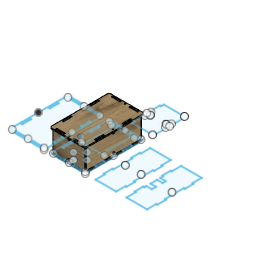
final l final v1 (Autodesk Fusion 360 design; units mm, degrees)
Autodesk Fusion 360 part; units mm, degrees
sketch "Sketch1" plane through (0, 0, 0) normal (0, 0, 1) x (1, 0, 0)
  line L0 (180, 78.114) -> (177.2, 78.114)
  line L1 (90, 52.114) -> (90, 78.114)
  line L2 (90, 81.114) -> (90, 107.114)
  line L3 (177.2, 76.484) -> (174.45, 76.484)
  line L4 (-89.654, 3.2) -> (-89.654, 6.6)
  line L5 (84.45, 76.484) -> (84.45, 78.114)
  arc A0 (-5, 0) -> (0, 5) centre (-5, 5) ccw
  line L6 (-64.654, 6.6) -> (-64.654, 3.2)
  line L7 (180, 0) -> (180, 27.114)
  line L8 (37, 78.114) -> (37, 79.614)
  line L9 (35.55, 76.484) -> (35.55, 78.114)
  line L10 (120, 27.114) -> (120, 0)
  line L11 (183.2, 52.114) -> (180, 52.114)
  circle A1 centre (-17.936, 73.3627) radius 1.5
  circle A2 centre (-4.7, 86.2139) radius 1.7
  line L12 (183.2, 27.114) -> (183.2, 52.114)
  line L13 (37, 81.114) -> (37, 79.614)
  line L14 (87.2, 76.484) -> (84.45, 76.484)
  line L15 (120, 57.814) -> (120, 52.114)
  line L16 (-97.872, 0) -> (-5, 0)
  line L17 (90, 81.114) -> (87.2, 81.114)
  line L18 (-5.55, 239.345) -> (-5.55, 240.975)
  line L19 (-2.8, 240.975) -> (-2.8, 239.345)
  line L20 (-2.8, 240.975) -> (-2.8, 239.345)
  line L21 (-38.218, 3.2) -> (-13.218, 3.2)
  line L22 (84.45, 78.114) -> (83, 78.114)
  line L23 (35.55, 81.114) -> (37, 81.114)
  line L24 (-5.55, 240.975) -> (-7, 240.975)
  line L25 (-96.472, 33.7139) -> (-99.872, 33.7139)
  line L26 (0, 233.518) -> (0, 240.975)
  line L27 (93.2, 52.114) -> (90, 52.114)
  line L28 (-3, 58.7139) -> (-3, 33.7139)
  line L29 (35.55, 78.114) -> (37, 78.114)
  line L30 (90, 0) -> (90, 27.114)
  line L31 (30, 27.114) -> (26.8, 27.114)
  line L32 (0, 240.975) -> (-2.8, 240.975)
  line L33 (26.8, 27.114) -> (26.8, 52.114)
  line L34 (-38.218, 6.6) -> (-38.218, 3.2)
  arc A3 (-102.872, 5) -> (-97.872, 0) centre (-97.872, 5) ccw
  line L35 (0, 240.975) -> (-2.8, 240.975)
  line L36 (0, 233.518) -> (0, 240.975)
  line L37 (93.2, 27.114) -> (93.2, 52.114)
  line L38 (3.2, 204.257) -> (0, 204.257)
  line L39 (32.8, 78.114) -> (32.8, 76.484)
  circle A4 centre (-51.436, 4.7) radius 1.7
  line L40 (-99.872, 58.7139) -> (-96.472, 58.7139)
  circle A5 centre (-51.436, 16.9336) radius 7
  line L41 (90, 27.114) -> (93.2, 27.114)
  circle A6 centre (-98.172, 86.2139) radius 1.7
  line L42 (87.2, 78.114) -> (87.2, 76.484)
  line L43 (83, 78.114) -> (83, 79.614)
  line L44 (120, 57.814) -> (136, 57.814)
  circle A7 centre (-71.436, 36.9336) radius 7
  line L45 (32.8, 76.484) -> (35.55, 76.484)
  line L46 (-77.936, 73.5127) -> (-24.936, 73.5127)
  line L47 (-64.654, 3.2) -> (-89.654, 3.2)
  circle A8 centre (-51.436, 56.9336) radius 7
  circle A9 centre (-84.936, 73.3627) radius 1.5
  line L48 (120, 89.314) -> (120, 69.914)
  line L49 (84.45, 82.744) -> (84.45, 81.114)
  line L50 (173, 81.114) -> (173, 79.614)
  line L51 (26.8, 52.114) -> (30, 52.114)
  line L52 (180, 81.114) -> (180, 107.114)
  line L53 (35.55, 82.744) -> (35.55, 81.114)
  line L54 (32.8, 82.744) -> (35.55, 82.744)
  line L55 (-89.654, 6.6) -> (-64.654, 6.6)
  circle A10 centre (-31.436, 36.9336) radius 7
  line L56 (87.2, 82.744) -> (84.45, 82.744)
  line L57 (84.45, 81.114) -> (83, 81.114)
  line L58 (32.8, 81.114) -> (32.8, 82.744)
  line L59 (0, 229.257) -> (0, 233.518)
  line L60 (-96.472, 58.7139) -> (-96.472, 33.7139)
  line L61 (-6.4, 33.7139) -> (-6.4, 58.7139)
  line L62 (-5.55, 240.975) -> (-7, 240.975)
  line L63 (3.2, 229.257) -> (3.2, 204.257)
  line L64 (-3, 33.7139) -> (-6.4, 33.7139)
  line L65 (30, 78.114) -> (32.8, 78.114)
  line L66 (30, 78.114) -> (30, 52.114)
  line L67 (-2.8, 239.345) -> (-5.55, 239.345)
  line L68 (87.2, 81.114) -> (87.2, 82.744)
  line L69 (30, 27.114) -> (30, 0)
  line L70 (3.2, 229.257) -> (0, 229.257)
  line L71 (-13.218, 3.2) -> (-13.218, 6.6)
  line L72 (30, 81.114) -> (32.8, 81.114)
  line L73 (-5.55, 239.345) -> (-5.55, 240.975)
  line L74 (-6.4, 58.7139) -> (-3, 58.7139)
  line L75 (90, 78.114) -> (87.2, 78.114)
  line L76 (0, 196.039) -> (0, 204.257)
  line L77 (-13.218, 6.6) -> (-38.218, 6.6)
  line L78 (-2.8, 239.345) -> (-5.55, 239.345)
  line L79 (83, 81.114) -> (83, 79.614)
  line L80 (-99.872, 33.7139) -> (-99.872, 58.7139)
  line L81 (-38.218, 169.2277) -> (-13.218, 169.2277)
  line L82 (-2.8, 243.975) -> (-2.8, 245.605)
  line L83 (120, 107.114) -> (120, 98.314)
  circle A11 centre (-84.936, 160.6627) radius 1.5
  line L84 (120, 132.114) -> (116.8, 132.114)
  line L85 (93.2, 132.114) -> (93.2, 107.114)
  line L86 (180, 132.114) -> (180, 159.228)
  line L87 (0, 255.693) -> (0, 251.432)
  line L88 (-2.8, 243.975) -> (-2.8, 245.605)
  line L89 (116.8, 107.114) -> (120, 107.114)
  line L90 (-64.654, 169.2277) -> (-89.654, 169.2277)
  line L91 (90, 132.114) -> (90, 159.228)
  line L92 (26.8, 132.114) -> (26.8, 107.114)
  line L93 (93.2, 107.114) -> (90, 107.114)
  line L94 (120, 89.314) -> (136, 89.314)
  line L95 (-6.4, 113.7139) -> (-3, 113.7139)
  line L96 (-3, 138.7139) -> (-6.4, 138.7139)
  line L97 (-120, 5) -> (-120, 167.4277)
  line L98 (-64.654, 165.8277) -> (-64.654, 169.2277)
  line L99 (-3, 113.7139) -> (-3, 138.7139)
  line L100 (-222.872, 5) -> (-222.872, 167.4277)
  line L101 (-5.55, 245.605) -> (-5.55, 243.975)
  line L102 (-53, 243.975) -> (-53, 242.475)
  line L103 (-24.936, 160.5127) -> (-77.936, 160.5127)
  line L104 (3.2, 280.693) -> (0, 280.693)
  line L105 (180, 132.114) -> (183.2, 132.114)
  line L106 (-184.654, 3.2) -> (-209.654, 3.2)
  line L107 (120, 159.228) -> (120, 132.114)
  line L108 (116.8, 52.114) -> (120, 52.114)
  line L109 (0, 280.693) -> (0, 288.911)
  line L110 (0, 243.975) -> (-2.8, 243.975)
  line L111 (116.8, 132.114) -> (116.8, 107.114)
  line L112 (180, 159.228) -> (120, 159.228)
  line L113 (0, 243.975) -> (-2.8, 243.975)
  line L114 (183.2, 107.114) -> (180, 107.114)
  line L115 (0, 196.039) -> (-60, 196.039)
  line L116 (-38.218, 165.8277) -> (-38.218, 169.2277)
  line L117 (90, 132.114) -> (93.2, 132.114)
  line L118 (136, 98.314) -> (120, 98.314)
  line L119 (-60, 288.911) -> (0, 288.911)
  line L120 (26.8, 107.114) -> (30, 107.114)
  line L121 (-5.55, 245.605) -> (-5.55, 243.975)
  line L122 (90, 159.228) -> (30, 159.228)
  line L123 (-13.218, 169.2277) -> (-13.218, 165.8277)
  line L124 (3.2, 255.693) -> (0, 255.693)
  line L125 (30, 132.114) -> (26.8, 132.114)
  line L126 (30, 107.114) -> (30, 81.114)
  line L127 (0, 243.975) -> (0, 251.432)
  circle A12 centre (-17.936, 160.6627) radius 1.5
  line L128 (-97.872, 172.4277) -> (-5, 172.4277)
  line L129 (-96.472, 138.7139) -> (-99.872, 138.7139)
  line L130 (30, 0) -> (90, 0)
  line L131 (-5.55, 243.975) -> (-7, 243.975)
  line L132 (30, 159.228) -> (30, 132.114)
  line L133 (-99.872, 138.7139) -> (-99.872, 113.7139)
  line L134 (120, 27.114) -> (116.8, 27.114)
  line L135 (-7, 243.975) -> (-7, 242.475)
  line L136 (-53, 240.975) -> (-53, 242.475)
  line L137 (-217.872, 0) -> (-125, 0)
  line L138 (177.2, 78.114) -> (177.2, 76.484)
  line L139 (-6.4, 138.7139) -> (-6.4, 113.7139)
  line L140 (-60, 196.039) -> (-60, 204.257)
  line L141 (-57.2, 245.605) -> (-54.45, 245.605)
  arc A13 (-97.872, 172.4277) -> (-102.872, 167.4277) centre (-97.872, 167.4277) ccw
  line L142 (-123, 58.7139) -> (-123, 33.7139)
  line L143 (-217.872, 172.4277) -> (-125, 172.4277)
  line L144 (-219.872, 138.7139) -> (-219.872, 113.7139)
  line L145 (183.2, 132.114) -> (183.2, 107.114)
  line L146 (-102.872, 5) -> (-102.872, 167.4277)
  line L147 (-60, 240.975) -> (-57.2, 240.975)
  line L148 (-184.654, 165.8277) -> (-184.654, 169.2277)
  line L149 (-63.2, 229.257) -> (-63.2, 204.257)
  line L150 (-126.4, 58.7139) -> (-123, 58.7139)
  line L151 (-7, 240.975) -> (-7, 242.475)
  line L152 (-219.872, 113.7139) -> (-216.472, 113.7139)
  circle A14 centre (-51.436, 167.7277) radius 1.7
  line L153 (3.2, 255.693) -> (3.2, 280.693)
  line L154 (-2.8, 245.605) -> (-5.55, 245.605)
  line L155 (-7, 240.975) -> (-7, 242.475)
  line L156 (-63.2, 229.257) -> (-60, 229.257)
  line L157 (-54.45, 240.975) -> (-53, 240.975)
  line L158 (-126.4, 33.7139) -> (-126.4, 58.7139)
  line L159 (-133.218, 3.2) -> (-133.218, 6.6)
  line L160 (-219.872, 58.7139) -> (-216.472, 58.7139)
  line L161 (-209.654, 165.8277) -> (-184.654, 165.8277)
  line L162 (-7, 243.975) -> (-7, 242.475)
  line L163 (-133.218, 165.8277) -> (-158.218, 165.8277)
  line L164 (-53, 240.975) -> (-53, 242.475)
  arc A15 (-125, 0) -> (-120, 5) centre (-125, 5) ccw
  line L165 (-54.45, 240.975) -> (-53, 240.975)
  line L166 (-2.8, 245.605) -> (-5.55, 245.605)
  line L167 (-123, 33.7139) -> (-126.4, 33.7139)
  line L168 (-63.2, 204.257) -> (-60, 204.257)
  line L169 (-133.218, 169.2277) -> (-133.218, 165.8277)
  line L170 (136, 89.314) -> (136, 98.314)
  line L171 (0, 243.975) -> (0, 251.432)
  line L172 (-123, 113.7139) -> (-123, 138.7139)
  line L173 (-216.472, 58.7139) -> (-216.472, 33.7139)
  line L174 (-13.218, 165.8277) -> (-38.218, 165.8277)
  line L175 (-53, 243.975) -> (-53, 242.475)
  line L176 (-99.872, 113.7139) -> (-96.472, 113.7139)
  arc A16 (0, 167.4277) -> (-5, 172.4277) centre (-5, 167.4277) ccw
  line L177 (0, 5) -> (0, 167.4277)
  line L178 (-54.45, 239.345) -> (-54.45, 240.975)
  line L179 (180, 52.114) -> (180, 78.114)
  line L180 (-5.55, 243.975) -> (-7, 243.975)
  line L181 (-89.654, 165.8277) -> (-64.654, 165.8277)
  line L182 (174.45, 82.744) -> (174.45, 81.114)
  line L183 (-209.654, 3.2) -> (-209.654, 6.6)
  line L184 (-60, 233.518) -> (-60, 240.975)
  line L185 (-158.218, 169.2277) -> (-133.218, 169.2277)
  line L186 (-54.45, 243.975) -> (-53, 243.975)
  line L187 (-209.654, 6.6) -> (-184.654, 6.6)
  line L188 (-60, 243.975) -> (-57.2, 243.975)
  line L189 (-126.4, 113.7139) -> (-123, 113.7139)
  line L190 (-158.218, 3.2) -> (-133.218, 3.2)
  line L191 (-54.45, 245.605) -> (-54.45, 243.975)
  line L192 (174.45, 78.114) -> (173, 78.114)
  line L193 (-77.936, 160.5127) -> (-77.936, 73.5127)
  line L194 (-57.2, 240.975) -> (-57.2, 239.345)
  line L195 (-219.872, 33.7139) -> (-219.872, 58.7139)
  arc A17 (-120, 167.4277) -> (-125, 172.4277) centre (-125, 167.4277) ccw
  line L196 (-184.654, 6.6) -> (-184.654, 3.2)
  arc A18 (-222.872, 5) -> (-217.872, 0) centre (-217.872, 5) ccw
  line L197 (-123, 138.7139) -> (-126.4, 138.7139)
  line L198 (-60, 240.975) -> (-57.2, 240.975)
  line L199 (-216.472, 33.7139) -> (-219.872, 33.7139)
  line L200 (-60, 243.975) -> (-60, 251.432)
  line L201 (-133.218, 6.6) -> (-158.218, 6.6)
  line L202 (-60, 243.975) -> (-60, 251.432)
  line L203 (116.8, 27.114) -> (116.8, 52.114)
  line L204 (-216.472, 138.7139) -> (-219.872, 138.7139)
  line L205 (-60, 229.257) -> (-60, 233.518)
  line L206 (180, 81.114) -> (177.2, 81.114)
  line L207 (136, 69.914) -> (120, 69.914)
  line L208 (-57.2, 243.975) -> (-57.2, 245.605)
  line L209 (-209.654, 169.2277) -> (-209.654, 165.8277)
  line L210 (136, 57.814) -> (136, 69.914)
  line L211 (-96.472, 113.7139) -> (-96.472, 138.7139)
  line L212 (180, 27.114) -> (183.2, 27.114)
  line L213 (-158.218, 165.8277) -> (-158.218, 169.2277)
  line L214 (-89.654, 169.2277) -> (-89.654, 165.8277)
  line L215 (-57.2, 239.345) -> (-54.45, 239.345)
  line L216 (-57.2, 243.975) -> (-57.2, 245.605)
  line L217 (-216.472, 113.7139) -> (-216.472, 138.7139)
  line L218 (-54.45, 239.345) -> (-54.45, 240.975)
  line L219 (-60, 255.693) -> (-60, 251.432)
  line L220 (-57.2, 239.345) -> (-54.45, 239.345)
  line L221 (177.2, 81.114) -> (177.2, 82.744)
  line L222 (173, 78.114) -> (173, 79.614)
  line L223 (-63.2, 255.693) -> (-63.2, 280.693)
  circle A19 centre (-124.7, 86.2139) radius 1.7
  line L224 (-24.936, 73.5127) -> (-24.936, 160.5127)
  line L225 (-57.2, 240.975) -> (-57.2, 239.345)
  line L226 (-63.2, 255.693) -> (-60, 255.693)
  line L227 (-158.218, 6.6) -> (-158.218, 3.2)
  circle A20 centre (-171.436, 4.7) radius 1.7
  line L228 (-60, 233.518) -> (-60, 240.975)
  line L229 (-54.45, 245.605) -> (-54.45, 243.975)
  line L230 (-54.45, 243.975) -> (-53, 243.975)
  line L231 (-63.2, 280.693) -> (-60, 280.693)
  line L232 (-60, 280.693) -> (-60, 288.911)
  line L233 (-57.2, 245.605) -> (-54.45, 245.605)
  line L234 (177.2, 82.744) -> (174.45, 82.744)
  line L235 (120, 0) -> (180, 0)
  line L236 (-60, 243.975) -> (-57.2, 243.975)
  line L237 (174.45, 81.114) -> (173, 81.114)
  line L238 (-184.654, 169.2277) -> (-209.654, 169.2277)
  line L239 (-126.4, 138.7139) -> (-126.4, 113.7139)
  circle A21 centre (-171.436, 167.7277) radius 1.7
  line L240 (174.45, 76.484) -> (174.45, 78.114)
  arc A22 (-217.872, 172.4277) -> (-222.872, 167.4277) centre (-217.872, 167.4277) ccw
  point P0 (-84.936, 73.3627)
  point P1 (-102.872, 86.2139)
  point P2 (-51.436, 16.9336)
  point P3 (-120, 0)
  point P4 (-222.872, 86.2139)
  point P5 (-63.2, 242.475)
  point P6 (3.2, 242.475)
  dimension "d14" = 25
  dimension "d185" = 14
  dimension "d187" = 14
  dimension "d191" = 14
  dimension "d192" = 14
  dimension "d197" = 3
  dimension "d198" = 53
  dimension "d199" = 87
  dimension "d209" = 25
  dimension "d210" = 3.2
  dimension "d213" = 25
  dimension "d214" = 3.2
  dimension "d219" = 60
  dimension "d220" = 159.228
  dimension "d221" = 27.114
  dimension "d222" = 3.2
  dimension "d223" = 25
  dimension "d225" = 2.8
  dimension "d226" = 1.63
  dimension "d227" = 2.75
  dimension "d228" = 1.45
  dimension "d234" = 2.8
  dimension "d235" = 1.63
  dimension "d236" = 2.75
  dimension "d237" = 1.45
  dimension "d238" = 60
  dimension "d239" = 159.228
  dimension "d240" = 27.114
  dimension "d241" = 3.2
  dimension "d242" = 25
  dimension "d252" = 2.8
  dimension "d253" = 1.63
  dimension "d254" = 2.75
  dimension "d255" = 1.45
  dimension "d256" = 25
  dimension "d265" = 25
  dimension "d266" = 3.2
  dimension "d267" = 25
  dimension "d268" = 3.2
  dimension "d288" = 5
  dimension "d289" = 5
  dimension "d290" = 5
  dimension "d292" = 12.1
  dimension "d293" = 19.4
  dimension "d294" = 9
  dimension "d296" = 26.436
  dimension "d297" = 13.218
  dimension "d298" = 13.218
  dimension "d299" = 25
  dimension "d300" = 25
  dimension "d301" = 92.872
  dimension "d303" = 92.872
  constraint horizontal L16
  constraint horizontal L25
  constraint vertical L80
  constraint horizontal L40
  constraint vertical L60
  constraint horizontal L46
  constraint perpendicular L46 L224
  constraint parallel L46 L103
  constraint parallel L193 L224
  constraint perpendicular L128 L146
  constraint perpendicular L128 L177
  constraint horizontal L64
  constraint vertical L61
  constraint horizontal L74
  constraint vertical L28
  constraint horizontal L130
  constraint vertical L30
  constraint horizontal L122
  constraint vertical L132
  constraint perpendicular L125 L132
  constraint perpendicular L92 L125
  constraint coincident L120.end L132
  constraint perpendicular L120 L132
  constraint collinear L30 L91
  constraint collinear L1 L30
  constraint collinear L1 L2
  constraint collinear L184 L200
  constraint horizontal L235
  constraint vertical L7
  constraint horizontal L112
  constraint vertical L107
  constraint perpendicular L84 L107
  constraint perpendicular L84 L111
  constraint coincident L83.start L107
  constraint perpendicular L89 L107
  constraint collinear L7 L86
  constraint collinear L7 L179
  constraint collinear L52 L179
  constraint collinear L202 L228
  constraint horizontal L137
  constraint horizontal L199
  constraint vertical L195
  constraint horizontal L160
  constraint vertical L173
  constraint perpendicular L100 L143
  constraint perpendicular L97 L143
  constraint horizontal L167
  constraint vertical L158
  constraint horizontal L150
  constraint vertical L142
  constraint tangent A16 L177
  constraint tangent L128 A16
  constraint coincident P1 L146
  constraint tangent A13 L146
  constraint tangent L128 A13
  constraint tangent L16 A3
  constraint tangent A3 L146
  constraint equal A3 A13
  constraint tangent A0 L177
  constraint tangent A0 L16
  constraint equal A0 A13
  constraint coincident P4 L100
  constraint tangent L100 A18
  constraint tangent L137 A18
  constraint equal A13 A18
  constraint tangent L97 A15
  constraint tangent L137 A15
  constraint equal A13 A15
  constraint tangent L100 A22
  constraint tangent L143 A22
  constraint equal A13 A22
  constraint tangent L97 A17
  constraint tangent L143 A17
  constraint perpendicular L44 L210
  constraint perpendicular L72 L126
  constraint perpendicular L83 L118
  constraint perpendicular L156 L228
  constraint perpendicular L223 L226
  constraint perpendicular L149 L156
  constraint perpendicular L149 L168
  constraint perpendicular L140 L168
  constraint perpendicular L223 L231
  measures "d14" distance of L25.start L40.end
  measures "d185" diameter of A8
  measures "d187" diameter of A5
  measures "d191" diameter of A10
  measures "d192" diameter of A7
  measures "d197" diameter of A11
  measures "d198" distance of L103.end L103.start
  measures "d199" distance of L46.end L103.start
  measures "d209" distance of L28.end L28.start
  measures "d213" distance of L4.start L6.end
  measures "d219" distance of L30.start L69.end
  measures "d220" distance of L69.end L122.end
  measures "d221" distance of L122.end L125.start
  measures "d222" distance of L92.start L125.start
  measures "d223" distance of L92.end L92.start
  measures "d225" distance of L65.start L39.start
  measures "d226" distance of L39.end L39.start
  measures "d227" distance of L9.start L39.end
  measures "d228" distance of L9.end L8.start
  measures "d234" distance of L147.start L147.end
  measures "d235" distance of L147.end L194.end
  measures "d236" distance of L178.start L194.end
  measures "d237" distance of L136.start L157.start
  measures "d238" distance of L7.start L10.end
  measures "d239" distance of L107.start L10.end
  measures "d240" distance of L84.start L107.start
  measures "d241" distance of L84.start L84.end
  measures "d242" distance of L84.end L89.start
  measures "d252" distance of L147.start L147.end
  measures "d253" distance of L194.end L147.end
  measures "d254" distance of L194.end L178.start
  measures "d255" distance of L157.start L136.start
  measures "d256" distance of L173.end L160.end
  measures "d265" distance of L142.start L142.end
  measures "d267" distance of L106.end L106.start
  measures "d288" radius of A16
  measures "d289" radius of A13
  measures "d290" radius of A17
  measures "d292" distance of L207.start L44.end
  measures "d293" distance of L48.start L48.end
  measures "d294" distance of L118.start L94.end
  measures "d296" distance of L98 L116
  measures "d297" distance of L149.start P5
  measures "d298" distance of L223.start P5
  measures "d299" distance of L223.start L223.end
  measures "d300" distance of L149.start L149.end
  measures "d301" distance of L143.start L143.end
  measures "d303" distance of L109.end L76.start
extrude "Extrude1" add sketch "Sketch1" along normal blind 3.2 contours L18 L19 L20 L24 L26 L32 L35 L36 L38 L59 L62 L63 L67 L70 L73 L76 L78 L82 L87 L88 L101 L102 L104 L109 L110 L113 L115 L119 L121 L124 L127 L131 L135 L136 L140 L141 L147 L149 L151 L153 L154 L155 L156 L157 L162 L164 L165 L166 L168 L171 L175 L178 L180 L184 L186 L188 L191 L194 L198 L200 L202 L205 L208 L215 L216 L218 L219 L220 L223 L225 L226 L228 L229 L230 L231 L232 L233 L236 makes body 1 in component "Component"
extrude "Extrude1'" add sketch "Sketch1" along normal blind 3.2 separate body contours L97 L100 L137 L143 A15 A17 A18 A22 makes body 2 in component "Component'"
extrude "Extrude1''" add sketch "Sketch1" along normal blind 3.2 separate body contours L18 L19 L20 L24 L26 L32 L35 L36 L38 L59 L62 L63 L67 L70 L73 L76 L78 L82 L87 L88 L101 L102 L104 L109 L110 L113 L115 L119 L121 L124 L127 L131 L135 L136 L140 L141 L147 L149 L151 L153 L154 L155 L156 L157 L162 L164 L165 L166 L168 L171 L175 L178 L180 L184 L186 L188 L191 L194 L198 L200 L202 L205 L208 L215 L216 L218 L219 L220 L223 L225 L226 L228 L229 L230 L231 L232 L233 L236 makes body 3 in component "Component''"
extrude "Extrude1'''" add sketch "Sketch1" along normal blind 3.2 separate body contours A0 L16 A3 L128 A13 L146 A16 L177 makes body 4 in component "Component'''"
extrude "Extrude1''''" add sketch "Sketch1" along normal blind 3.2 separate body contours L1 L2 L5 L8 L9 L13 L14 L17 L22 L23 L27 L29 L30 L31 L33 L37 L39 L41 L42 L43 L45 L49 L51 L53 L54 L56 L57 L58 L65 L66 L68 L69 L72 L75 L79 L85 L91 L92 L93 L117 L120 L122 L125 L126 L130 L132 makes body 5 in component "Component''''"
extrude "Extrude1'''''" add sketch "Sketch1" along normal blind 3.2 separate body contours L0 L3 L7 L10 L11 L12 L15 L44 L48 L50 L52 L83 L84 L86 L89 L94 L105 L107 L108 L111 L112 L114 L118 L134 L138 L145 L170 L179 L182 L192 L203 L206 L207 L210 L212 L221 L222 L234 L235 L237 L240 makes body 6 in component "Component'''''"
component "Component" placed x (0, 0, -1) y (1, 0, 0) z (0, -1, 0) at (-293.911, 168.8277, 3.2)
component "Component'" placed x (1, 0, 0) y (0, 1, 0) z (0, 0, 1) at (120, -0.4, 63.4)
component "Component''" placed x (0, 0, 1) y (-1, 0, 0) z (0, -1, 0) at (191.039, 6.6, 63.2)
component "Component'''" placed x (1, 0, 0) y (0, 1, 0) z (0, 0, 1) at (0, 0, 0)
component "Component''''" placed x (0, 0, 1) y (0, 1, 0) z (-1, 0, 0) at (-3.2, 6.1999, -26.6)
component "Component'''''" placed x (0, 0, -1) y (0, -1, 0) z (-1, 0, 0) at (-96.672, 165.4279, 183.4)
equation "d210 = t"
equation "d214 = t"
equation "d266 = t"
equation "d268 = t"
equation "d297 = 26.436024 mm / 2"
equation "d298 = 26.436024 mm / 2"
equation "t = 3.2 mm"
equation "d55 = t"
equation "d57 = t"
equation "d55_1 = t"
equation "d63 = t"
equation "d77 = t"
equation "d79 = t"
